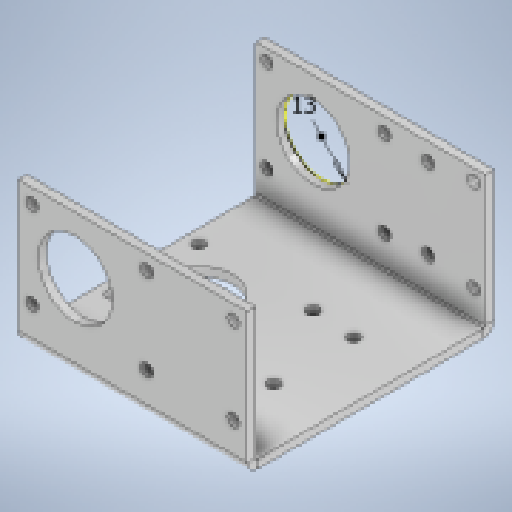
# Autodesk Inventor part: axis_20_bottom_frame
Saved by Autodesk Inventor 2025.2 (Build 292293000, 293)
## iProperties
Created: 2025-05-07
Part Number: axis_20_bottom_frame
Material: Aluminum 6061-AHC
Document SubType Name: Sheet Metal
Designer: LG
Density: 2.7 g/cm^3
Sheet Metal Rule: Default_mm
Appearance: Aluminum - Dark
Author: LG
Autodesk Inventor part; units mm, degrees
ref_plane "YZ Plane" through (0, 0, 0) normal (1, 0, 0) x (0, 1, 0)
ref_plane "XZ Plane" through (0, 0, 0) normal (0, 1, 0) x (-1, 0, 0)
ref_plane "XY Plane" through (0, 0, 0) normal (0, 0, 1) x (1, 0, 0)
sketch "Sketch1" plane through (0, 0, 0) normal (0, 1, 0) x (-1, 0, 0)
  line L0 (-20, 20) -> (20, 20)
  line L1 (20, 20) -> (20, -20)
  line L2 (20, -20) -> (-20, -20)
  line L3 (-20, -20) -> (-20, 20)
  line L4 (-20, 20) -> (20, -20) construction
  line L5 (20, 20) -> (-20, -20) construction
  point P0 (0, 0)
  dimension "d0" = 40
  dimension "d1" = 40
  measures "d0" distance of L0.end L1.end
  measures "d1" distance of L1.end L2.end
extrude "Plate1" add sketch "Sketch1" along normal blind 1.5
sketch "Sketch2" plane through (20, 0, 21.5) normal (0, 0, -1) x (-1, 0, 0)
  line L0 (40, 0) -> (0, 0)
  line L1 (0, 0) -> (0, 24.64)
  line L2 (0, 24.64) -> (40, 24.64)
  line L3 (40, 24.64) -> (40, 0)
  constraints: 8 end point
edge flange "Flange1" height 24.64 angle 90 thickness 1.5 bend radius 0.31 thickness toward (0, 0, -1) relief straight relief width 1.5 relief depth 0.75 corner gap 0.31 corner form 0 edges at (0, 1.5, 20) (0, 1.5, -20) wall of the first edge with corners at (-20, 0, 21.5) (20, 0, 21.5) (20, 24.64, 21.5) (-20, 24.64, 21.5)
bend "Bend1"
corner "Corner1"
sketch "Sketch3" plane through (20, 24.64, -21.5) normal (0, 0, -1) x (-1, 0, 0)
  circle A0 centre (30.05, -10.07) radius 6.4 projected
  point P0 (20, -24.64)
extrude "Cut1" cut sketch "Sketch3" against normal blind 1.5
sketch "Sketch4" plane through (20, 24.64, -21.5) normal (0, 0, -1) x (-1, 0, 0)
  circle A0 centre (9.93, -3.07) radius 0.7835 projected
  circle A1 centre (38.05, -2) radius 0.7835 projected
  circle A2 centre (9.93, -17.07) radius 0.7835 projected
  circle A3 centre (1.95, -2) radius 0.7835 projected
  circle A4 centre (1.95, -18.14) radius 0.7835 projected
  circle A5 centre (38.05, -18.14) radius 0.7835 projected
  point P0 (20, -24.64)
hole "Hole1" at (18.05, 22.64, -21.5) at (10.07, 21.57, -21.5) at (18.05, 6.5, -21.5) at (10.07, 7.57, -21.5) at (-18.05, 6.5, -21.5) at (-18.05, 22.64, -21.5) direction (0, 0, 1) diameter 2.1 depth 1.5
sketch "Sketch5" plane through (-20, 24.64, 21.5) normal (0, 0, 1) x (1, 0, 0)
  circle A0 centre (9.95, -10.07) radius 6 projected
  point P0 (20, -24.64)
extrude "Cut2" cut sketch "Sketch5" against normal blind 1.5
sketch "Sketch6" plane through (-20, 24.64, 21.5) normal (0, 0, 1) x (1, 0, 0)
  circle A0 centre (2.45, -2.545) radius 0.7835 projected
  circle A1 centre (2.45, -17.595) radius 0.7835 projected
  circle A2 centre (37.55, -2.545) radius 0.7835 projected
  circle A3 centre (37.55, -17.595) radius 0.7835 projected
  circle A4 centre (22.45, -17.595) radius 0.7835 projected
  circle A5 centre (22.45, -2.545) radius 0.7835 projected
  point P0 (20, -24.64)
hole "Hole2" at (-17.55, 22.095, 21.5) at (2.45, 22.095, 21.5) at (17.55, 22.095, 21.5) at (17.55, 7.045, 21.5) at (2.45, 7.045, 21.5) at (-17.55, 7.045, 21.5) direction (0, 0, -1) diameter 2.1 depth 1.5
sketch "Sketch7" plane through (0, 1.5, 0) normal (0, 1, 0) x (1, 0, 0)
  circle A0 centre (10.07, 7) radius 0.7835 projected
  circle A1 centre (10.07, -7) radius 0.7835 projected
  circle A2 centre (-17.55, 7.525) radius 0.7835 projected
  circle A3 centre (-17.55, -7.525) radius 0.7835 projected
  circle A4 centre (2.45, -7.525) radius 0.7835 projected
  circle A5 centre (2.45, 7.525) radius 0.7835 projected
  point P0 (0, 0)
hole "Hole3" at (-17.55, 1.5, 7.525) at (-17.55, 1.5, -7.525) at (2.45, 1.5, -7.525) at (2.45, 1.5, 7.525) at (10.07, 1.5, 7) at (10.07, 1.5, -7) direction (0, -1, 0) diameter 2.1 depth 1.5
sketch "Sketch8" plane through (0, 1.5, 0) normal (0, 1, 0) x (1, 0, 0)
  circle A0 centre (-10.05, 0) radius 6 projected
  point P0 (0, 0)
extrude "Cut3" cut sketch "Sketch8" against normal blind 1.5
sketch "Sketch9" plane through (20, 24.64, -21.5) normal (0, 0, -1) x (-1, 0, 0)
  circle A0 centre (17.55, -2.545) radius 1.05 projected
  circle A1 centre (17.55, -17.595) radius 0.7835 projected
  point P0 (20, -24.64)
hole "Hole4" at (2.45, 22.095, -21.5) at (2.45, 7.045, -21.5) direction (0, 0, 1) diameter 2.1 depth 1.5
sketch "Sketch10" plane through (-20, 24.64, 21.5) normal (0, 0, 1) x (1, 0, 0)
  circle A0 centre (9.95, -10.07) radius 6.5
  circle A1 centre (9.95, -10.07) radius 6 projected
  point P0 (20, -24.64)
  dimension "d47" = 13
  constraints: 1 centre point, 1 concentric
  measures "d47" diameter of A0
extrude "Cut4" cut sketch "Sketch10" against normal blind 1.5 contours A0 | A1
sketch "Sketch12" plane through (0, 0, 0) normal (0, -1, 0) x (1, 0, 0)
  circle A0 centre (-10.05, 0) radius 6.5
  circle A1 centre (-10.05, 0) radius 6 projected
  point P0 (0, 0)
  dimension "d51" = 13
  constraints: 1 centre point, 1 concentric
  measures "d51" diameter of A0
extrude "Cut5" cut sketch "Sketch12" against normal blind 1.5 contours A0 | A1
equation "\"d13\" = Thickness"
equation "\"d20\" = Thickness"
equation "\"d22\" = Thickness"
equation "\"d29\" = Thickness"
equation "\"d36\" = Thickness"
equation "\"d38\" = Thickness"
equation "\"d45\" = Thickness"
equation "\"d48\" = Thickness"
equation "\"d52\" = Thickness"
equation "\"d2\" = Thickness"
equation "\"d3\" = BendReliefWidth"
equation "\"d4\" = BendReliefDepth"
equation "\"d5\" = MinimumRemnant"
equation "\"d6\" = TransitionRadius"
equation "\"d9\" = BendRadius"
equation "\"d10\" = CornerReliefSize"
equation "\"d11\" = GapSize"
equation "\"d12\" = JacobiRadiusSize"
equation "\"BendReliefWidth\" = Thickness"
equation "\"BendReliefDepth\" = 0.5 * Thickness"
equation "\"CornerReliefSize\" = 4 * Thickness"
equation "\"MinimumRemnant\" = 2 * Thickness"
equation "\"TransitionRadius\" = BendRadius"
equation "\"JacobiRadiusSize\" = BendRadius"
equation "\"GapSize\" = Thickness"
equation "\"Thickness\" = 1.5"
equation "\"BendRadius\" = 0.31"
body "Solid1"
